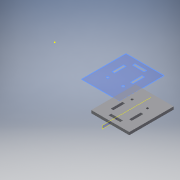
# Autodesk Inventor part: arm4_11
Saved by Autodesk Inventor 2016 (Build 200138000, 138)
## iProperties
Created: 2017-09-22
Part Number: arm4_11
Material: Generic
Document SubType Name: Modeling
Designer: student
Density: 1 g/cm^3
Appearance: Default
Author: student
Autodesk Inventor part; units mm, degrees
ref_plane "YZ Plane" through (0, 0, 0) normal (1, 0, 0) x (0, 1, 0)
ref_plane "XZ Plane" through (0, 0, 0) normal (0, 1, 0) x (-1, 0, 0)
ref_plane "XY Plane" through (0, 0, 0) normal (0, 0, 1) x (1, 0, 0)
sketch "Sketch1" plane through (0, 0, 0) normal (0, 1, 0) x (-1, 0, 0)
  arc A0 (-110.5448, 1.666) -> (-110.4284, 1.6651) centre (-110.4068, 11.3006) ccw construction
  arc A1 (-94.0784, 1.6651) -> (-94.0348, 1.6644) centre (-93.8968, 11.3006) ccw construction
  circle A2 centre (-110.4068, 11.3006) radius 1.143
  circle A3 centre (-93.8968, 11.3006) radius 1.143
  line L0 (-108.2859, -8.1857) -> (-96.2209, -8.1857) construction
  line L1 (-102.2534, 42.9953) -> (-122.5734, 42.9953)
  line L2 (-102.2534, 42.9953) -> (-81.9334, 42.9953)
  line L3 (-122.5734, 42.9953) -> (-122.5734, -4.3774)
  line L4 (-122.5734, -4.3774) -> (-81.9334, -4.3774)
  line L5 (-81.9334, -4.3774) -> (-81.9334, 42.9953)
  line L6 (-89.5534, -4.3774) -> (-114.9534, -4.3774) construction
  line L7 (-96.0304, 38.4741) -> (-108.4764, 38.4741)
  line L8 (-108.4764, 38.4741) -> (-108.4764, 35.7563)
  line L9 (-108.4764, 35.7563) -> (-96.0304, 35.7563)
  line L10 (-96.0304, 35.7563) -> (-96.0304, 38.4741)
  line L11 (-113.4226, 18.8009) -> (-110.7048, 18.8009)
  line L12 (-110.7048, 18.8009) -> (-110.7048, 31.2469)
  line L13 (-110.7048, 31.2469) -> (-113.4226, 31.2469)
  line L14 (-113.4226, 31.2469) -> (-113.4226, 18.8009)
  line L15 (-91.0842, 18.8009) -> (-93.802, 18.8009)
  line L16 (-93.802, 18.8009) -> (-93.802, 31.2469)
  line L17 (-93.802, 31.2469) -> (-91.0842, 31.2469)
  line L18 (-91.0842, 31.2469) -> (-91.0842, 18.8009)
  arc A4 (-93.8968, 10.028) -> (-93.9768, 12.5706) centre (-93.8968, 11.3006) ccw construction
  arc A5 (-110.3268, 12.5706) -> (-110.4068, 10.028) centre (-110.4068, 11.3006) ccw construction
  line L19 (-109.7718, 18.8653) -> (-94.5318, 18.8653) construction
  line L20 (-91.008, 15.4989) -> (-91.008, 18.6739) construction
  line L21 (-92.4431, 31.2469) -> (-92.4431, 18.8009) construction
  line L22 (-91.0842, 25.0239) -> (-93.802, 25.0239) construction
  line L23 (-112.0637, 18.8009) -> (-112.0637, 31.2469) construction
  line L24 (-110.7048, 25.0239) -> (-113.4226, 25.0239) construction
  line L25 (-96.0304, 37.1152) -> (-108.4764, 37.1152) construction
  line L26 (-102.2534, 35.7563) -> (-102.2534, 38.4741) construction
  point P0 (0, 0)
  point P1 (-102.2534, 36.3575)
  dimension "d0" = 2.286
  dimension "d1" = 2.286
  dimension "d19" = 3.175
  dimension "d23" = 6.223
  dimension "d24" = 1.3589
  dimension "d25" = 6.223
  dimension "d26" = 1.3589
  dimension "d27" = 6.223
  dimension "d28" = 1.3589
  constraints: 52 end point, 12 midpoint, 8 point on circle, 7 horizontal, 6 centre point, 4 parallel, 4 perpendicular, 4 vertical, 2 coincident, 8 other
  measures "d0" diameter of A2
  measures "d1" diameter of A3
  measures "d19" distance of L20.start L20.end
  measures "d23" distance between parallel lines of L22 L17
  measures "d24" distance between parallel lines of L21 L18
  measures "d25" distance between parallel lines of L26 L8
  measures "d26" distance between parallel lines of L25 L7
  measures "d27" distance between parallel lines of L24 L13
  measures "d28" distance between parallel lines of L23 L14
extrude "Extrusion1" add sketch "Sketch1" along normal blind 2.921
ref_plane "Work Plane1" through (102.2534, 0, 38.4741) normal (-1, 0, 0) x (0, 0, 1)
sketch "Sketch2" plane through (0, 2.921, 0) normal (0, 1, 0) x (1, 0, 0)
  point P0 (0, 0)
body "Solid1"
